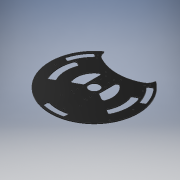
# Autodesk Inventor part: 2nd Plate
Saved by Autodesk Inventor 2017 (Build 210142000, 142)
## iProperties
Created: 2019-02-08
Part Number: 2nd Plate
Material: Generic
Document SubType Name: Modeling
Designer: cresswnd
Density: 1 g/cm^3
Appearance: Smooth - Black
Author: cresswnd
Autodesk Inventor part; units mm, degrees
ref_plane "YZ Plane" through (0, 0, 0) normal (1, 0, 0) x (0, 1, 0)
ref_plane "XZ Plane" through (0, 0, 0) normal (0, 1, 0) x (-1, 0, 0)
ref_plane "XY Plane" through (0, 0, 0) normal (0, 0, 1) x (1, 0, 0)
sketch "Sketch1" plane through (0, 0, 0) normal (0, 0, 1) x (1, 0, 0)
  circle A0 centre (21.75, 0.25) radius 1.45
  circle A1 centre (2.9989, 0.2602) radius 1.45
  circle A2 centre (-63.3205, 115.128) radius 1.45
  circle A3 centre (-53.9516, 131.369) radius 1.45
  circle A4 centre (78.6938, 131.3651) radius 1.45
  circle A5 centre (88.0766, 115.131) radius 1.45
  arc A6 (-37.626, 149.9172) -> (62.3772, 149.9149) centre (12.3777, 242.2475) ccw
  arc A7 (62.3772, 149.9149) -> (73.2296, 167.818) centre (52.5063, 168.1391) ccw
  arc A8 (-48.4787, 167.8183) -> (-37.626, 149.9172) centre (-27.7565, 168.1409) ccw
  arc A9 (-48.4787, 167.8183) -> (73.2296, 167.818) centre (12.3752, 82.2503) ccw
  circle A10 centre (12.3748, 82.2511) radius 100.0002 construction
  circle A11 centre (12.375, 82.2501) radius 12.5
  circle A12 centre (12.375, 82.2501) radius 87.5 construction
  line L0 (37.3748, -14.5737) -> (37.375, -1.6024) construction
  line L1 (-12.6233, -14.5742) -> (-12.6233, -1.603) construction
  line L2 (12.375, 82.2501) -> (114, 140.9233) construction
  line L3 (12.375, 82.2501) -> (-89.25, 140.9233) construction
  line L4 (108.7278, 109.0117) -> (97.4935, 102.5256) construction
  line L5 (83.7281, 152.3135) -> (72.4935, 145.827) construction
  arc A13 (108.7278, 109.0117) -> (83.7281, 152.3135) centre (12.3747, 82.2511) ccw
  arc A14 (97.4935, 102.5256) -> (72.4935, 145.827) centre (12.375, 82.2501) ccw
  line L6 (97.4935, 102.5256) -> (108.7278, 109.0117)
  line L7 (72.4935, 145.827) -> (83.7281, 152.3135)
  line L8 (37.3748, -14.5737) -> (37.375, -1.6024)
  line L9 (-12.6233, -14.5742) -> (-12.6233, -1.603)
  arc A15 (-12.6233, -14.5742) -> (37.3748, -14.5737) centre (12.3748, 82.2511) ccw
  arc A16 (-12.6233, -1.603) -> (37.375, -1.6024) centre (12.375, 82.2501) ccw
  line L10 (-58.9785, 152.3136) -> (-47.7434, 145.827) construction
  line L11 (-83.9782, 109.012) -> (-72.7435, 102.5256) construction
  line L12 (-72.7435, 102.5256) -> (-83.9782, 109.012)
  line L13 (-47.7434, 145.827) -> (-58.9785, 152.3136)
  arc A17 (-47.7434, 145.827) -> (-72.7435, 102.5256) centre (12.375, 82.2501) ccw
  arc A18 (-58.9785, 152.3136) -> (-83.9782, 109.012) centre (12.3717, 82.2529) ccw
  arc A19 (86.7944, 117.8432) -> (89.1811, 112.3417) centre (88.0766, 115.131) ccw
  arc A20 (76.8399, 133.7237) -> (80.4092, 128.9039) centre (78.6938, 131.3651) ccw
  arc A21 (-55.6661, 128.9072) -> (-52.0944, 133.725) centre (-53.9516, 131.369) ccw
  arc A22 (-64.4413, 112.3452) -> (-62.0519, 117.8466) centre (-63.3205, 115.128) ccw
  arc A23 (24.7176, 0.6894) -> (18.7605, -0.0012) centre (21.75, 0.25) ccw
  arc A24 (5.9875, -0.0016) -> (0.0284, 0.6799) centre (2.9989, 0.2602) ccw
  arc A25 (5.9875, -0.0016) -> (18.7605, -0.0012) centre (12.3717, 82.2529) ccw
  arc A26 (5.9875, -0.0016) -> (18.7605, -0.0012) centre (12.3717, 82.2529) ccw construction
  arc A27 (-42.373, 143.9641) -> (-52.0944, 133.725) centre (12.3717, 82.2529) ccw
  arc A28 (-36.0176, 149.0641) -> (-52.0944, 133.725) centre (12.3717, 82.2529) ccw construction
  arc A29 (-55.6661, 128.9072) -> (-62.0519, 117.8466) centre (12.3717, 82.2529) ccw
  arc A30 (-55.6661, 128.9072) -> (-62.0519, 117.8466) centre (12.3717, 82.2529) ccw construction
  arc A31 (76.8399, 133.7237) -> (67.1202, 143.9618) centre (12.3717, 82.2529) ccw
  arc A32 (76.8399, 133.7237) -> (60.7668, 149.0608) centre (12.3717, 82.2529) ccw construction
  arc A33 (86.7944, 117.8432) -> (80.4092, 128.9039) centre (12.3717, 82.2529) ccw
  arc A34 (24.7176, 0.6894) -> (89.1811, 112.3417) centre (12.3717, 82.2529) ccw construction
  arc A35 (86.7944, 117.8432) -> (80.4092, 128.9039) centre (12.3717, 82.2529) ccw construction
  line L14 (12.3717, 82.2529) -> (-95.0009, 20.2559) construction
  line L15 (12.3717, 82.2529) -> (12.3717, -55.9971) construction
  line L16 (12.3717, 82.2529) -> (116.9996, 21.845) construction
  arc A36 (-5.1266, 121.5334) -> (29.8753, 121.5311) centre (12.3717, 82.2529) ccw
  arc A37 (51.9253, 136.9246) -> (67.1202, 143.9618) centre (12.3752, 242.2457) ccw
  arc A38 (-42.373, 143.9641) -> (-27.1754, 136.9252) centre (12.3752, 242.2457) ccw
  line L17 (-23.6173, 58.5837) -> (-26.1173, 62.9138) construction
  line L18 (-26.1173, 62.9138) -> (-23.3483, 64.5125) construction
  line L19 (-23.6173, 58.5837) -> (-19.3458, 61.3318) construction
  line L20 (-23.5558, 58.6232) -> (2.0509, 58.6232) construction
  line L21 (-26.0543, 62.9502) -> (-3.8755, 75.7551)
  line L22 (-26.0543, 62.9502) -> (-0.4444, 62.9502) construction
  line L23 (12.3717, 82.2529) -> (-5.1266, 82.2529) construction
  line L24 (-5.1266, 82.2529) -> (-5.1266, 121.5334) construction
  line L25 (12.3717, 82.2529) -> (29.8753, 82.2529) construction
  line L26 (29.8753, 82.2529) -> (29.8753, 121.5311) construction
  line L27 (-5.1266, 82.2529) -> (-5.1266, 121.5334)
  line L28 (29.8753, 82.2529) -> (29.8753, 121.5311)
  line L29 (12.3717, 82.2529) -> (12.3717, 39.2511) construction
  line L30 (12.3717, 39.2511) -> (9.8717, 39.2511) construction
  line L31 (9.8717, 39.2511) -> (14.8717, 39.2511) construction
  line L32 (14.8717, 39.2511) -> (14.8717, 73.0001) construction
  line L33 (9.8717, 39.2511) -> (9.8717, 67.5643) construction
  line L34 (49.6122, 60.7517) -> (48.3622, 58.5867) construction
  line L35 (48.3622, 58.5867) -> (50.8622, 62.9168) construction
  line L36 (48.3622, 58.5867) -> (35.5366, 66.0323) construction
  line L37 (50.8622, 62.9168) -> (37.9999, 70.343) construction
  line L38 (50.7993, 62.9532) -> (28.6248, 75.7558)
  line L39 (3.3397, 3.2408) -> (3.3397, 15.3889)
  line L40 (3.3397, 3.2408) -> (15.4879, 3.2408) construction
  line L41 (21.4045, 3.23) -> (21.4045, 15.389)
  line L42 (21.4045, 3.23) -> (33.5635, 3.23) construction
  line L43 (-60.5689, 113.9329) -> (-50.0555, 107.863)
  line L44 (-60.5689, 113.9329) -> (-48.4291, 113.9329) construction
  line L45 (-51.5416, 129.5823) -> (-41.0226, 123.5092)
  line L46 (-51.5416, 129.5823) -> (-39.3953, 129.5823) construction
  line L47 (85.3244, 113.937) -> (74.8028, 107.8624)
  line L48 (85.3244, 113.937) -> (97.4738, 113.937) construction
  line L49 (76.2829, 129.5797) -> (65.7697, 123.5099)
  line L50 (76.2829, 129.5797) -> (88.4226, 129.5797) construction
  line L51 (-59.0714, 41.0016) -> (-57.8213, 38.8366) construction
  line L52 (-57.8213, 38.8366) -> (-60.3215, 43.1666) construction
  line L53 (-60.3215, 43.1666) -> (-52.3765, 47.7536) construction
  line L54 (-60.3215, 43.1666) -> (-51.1474, 43.1666) construction
  line L55 (-57.8213, 38.8366) -> (-51.421, 42.5318) construction
  line L56 (-57.8213, 38.8366) -> (-50.4308, 38.8366) construction
  line L57 (-57.7923, 38.8533) -> (-44.7683, 46.3728)
  line L58 (-57.7923, 38.8533) -> (-42.7534, 38.8533) construction
  line L59 (-60.2887, 43.1855) -> (-47.2728, 50.7003)
  line L60 (-60.2887, 43.1855) -> (-45.2593, 43.1855) construction
  line L61 (83.8121, 41.0061) -> (85.0621, 43.1712) construction
  line L62 (85.0621, 43.1712) -> (82.5621, 38.8411) construction
  line L63 (82.5621, 38.8411) -> (77.0249, 41.5028) construction
  line L64 (85.0621, 43.1712) -> (78.2875, 46.486) construction
  line L65 (82.5278, 38.8576) -> (69.5116, 46.3725)
  line L66 (82.5278, 38.8576) -> (97.5576, 38.8576) construction
  line L67 (85.0281, 43.1878) -> (72.0191, 50.6986)
  line L68 (85.0281, 43.1878) -> (100.0495, 43.1878) construction
  arc A39 (72.0191, 50.6986) -> (51.9253, 136.9246) centre (12.3717, 82.2529) ccw
  arc A40 (72.0191, 50.6986) -> (43.6909, 142.024) centre (12.3717, 82.2529) ccw construction
  arc A41 (24.7176, 0.6894) -> (82.5278, 38.8576) centre (12.3717, 82.2529) ccw
  arc A42 (85.0281, 43.1878) -> (89.1811, 112.3417) centre (12.3717, 82.2529) ccw
  arc A43 (-64.4413, 112.3452) -> (-60.2887, 43.1855) centre (12.3717, 82.2529) ccw construction
  arc A44 (-57.7923, 38.8533) -> (0.0284, 0.6799) centre (12.3717, 82.2529) ccw construction
  arc A45 (-64.4413, 112.3452) -> (-60.2887, 43.1855) centre (12.3717, 82.2529) ccw
  arc A46 (-57.7923, 38.8533) -> (0.0284, 0.6799) centre (12.3717, 82.2529) ccw
  arc A47 (-27.1754, 136.9252) -> (-47.2728, 50.7003) centre (12.3717, 82.2529) ccw
  arc A48 (-44.7683, 46.3728) -> (69.5116, 46.3725) centre (12.3717, 82.2529) ccw
  arc A49 (-5.1266, 82.2529) -> (-3.8755, 75.7551) centre (12.3717, 82.2529) ccw
  arc A50 (28.6248, 75.7558) -> (29.8753, 82.2529) centre (12.3717, 82.2529) ccw
  point P0 (-1.375, 71.4247)
  point P1 (9.8717, 39.3238)
  point P2 (9.8717, 64.9294)
  point P3 (14.8717, 39.3238)
  point P4 (14.8717, 64.9296)
  point P5 (48.2993, 58.6232)
  point P6 (26.1537, 71.4793)
  dimension "d0" = 25
  dimension "d1" = 175
  dimension "d15" = 6
  dimension "d16" = 6
  dimension "d17" = 6
  dimension "d18" = 6
  dimension "d19" = 6
  dimension "d20" = 6
  dimension "d31" = 5
  dimension "d33" = 30
  dimension "d34" = 2.5
  dimension "d35" = 5
  dimension "d36" = 2.5
  dimension "d37" = 5
  dimension "d38" = 90
  dimension "d39" = 90
  dimension "d40" = 30
  dimension "d41" = 30
  dimension "d42" = 150
  dimension "d43" = 150
  dimension "d44" = 2.5
  dimension "d45" = 5
  dimension "d46" = 30
  dimension "d47" = 30
  dimension "d48" = 30
  dimension "d49" = 30
  dimension "d50" = 2.5
  dimension "d51" = 5
  dimension "d52" = 150
  dimension "d53" = 150
  constraints: 138 end point, 115 point on circle, 50 centre point, 22 point on line, 18 horizontal, 13 coincident, 13 equal length, 7 perpendicular, 6 collinear, 5 tangent, 3 vertical, 2 concentric, 1 parallel, 13 other
  measures "d0" diameter of A11
  measures "d1" diameter of A12
  measures "d15" diameter of A19
  measures "d16" diameter of A20
  measures "d17" diameter of A21
  measures "d18" diameter of A22
  measures "d19" diameter of A23
  measures "d20" diameter of A24
  measures "d31" distance of L17.start L17.end
  measures "d33" angle of L22 L21
  measures "d34" distance of L29.end L30.end
  measures "d35" distance of L30.end L31.end
  measures "d36" distance of L34.start L34.end
  measures "d37" distance of L34.end L35.end
  measures "d38" angle of L40 L39
  measures "d39" angle of L42 L41
  measures "d40" angle of L43 L44
  measures "d41" angle of L45 L46
  measures "d42" angle of L47 L48
  measures "d43" angle of L49 L50
  measures "d44" distance of L51.start L51.end
  measures "d45" distance of L51.end L52.end
  measures "d46" angle of L54 L53
  measures "d47" angle of L56 L55
  measures "d48" angle of L58 L57
  measures "d49" angle of L60 L59
  measures "d50" distance of L61.start L61.end
  measures "d51" distance of L61.end L62.end
  measures "d52" angle of L66 L65
  measures "d53" angle of L68 L67
extrude "Extrusion4" add sketch "Sketch1" along normal blind 2 contours A6 A7 A9 A8 | A19 L47 A39 L49 A20 A33 | A21 L45 A47 L43 A22 A29 | A23 A25 A24 L39 A48 L41
fillet "Fillet1" radius 5 6 edges at (28.6248, 75.7558, 1) (50.7993, 62.9532, 1) (29.8753, 121.5311, 1) (-5.1266, 121.5334, 1) (-3.8755, 75.7551, 1) (-26.0543, 62.9502, 1)
fillet "Fillet2" radius 2 30 edges at (-51.5416, 129.5823, 1) (-52.0944, 133.725, 1) (-42.373, 143.9641, 1) (-27.1754, 136.9252, 1) (-41.0226, 123.5092, 1) (51.9253, 136.9246, 1) (67.1202, 143.9618, 1) (76.8399, 133.7237, 1) (76.2829, 129.5797, 1) (65.7697, 123.5099, 1) (89.1811, 112.3417, 1) (85.3244, 113.937, 1) (85.0281, 43.1878, 1) (72.0191, 50.6986, 1) (74.8028, 107.8624, 1) (21.4045, 15.389, 1) (21.4045, 3.23, 1) (24.7176, 0.6894, 1) (82.5278, 38.8576, 1) (69.5116, 46.3725, 1) (-60.5689, 113.9329, 1) (-64.4413, 112.3452, 1) (-50.0555, 107.863, 1) (-47.2728, 50.7003, 1) (-60.2887, 43.1855, 1) (-57.7923, 38.8533, 1) (-44.7683, 46.3728, 1) (3.3397, 3.2408, 1) (0.0284, 0.6799, 1) (3.3397, 15.3889, 1)
fillet "Fillet3" radius 3 12 edges at (37.3748, -14.5737, 1) (-12.6233, -14.5742, 1) (-12.6233, -1.603, 1) (37.375, -1.6024, 1) (-58.9785, 152.3136, 1) (-72.7435, 102.5256, 1) (-47.7434, 145.827, 1) (-83.9782, 109.012, 1) (72.4935, 145.827, 1) (83.7281, 152.3135, 1) (108.7278, 109.0117, 1) (97.4935, 102.5256, 1)
sketch "Sketch3" plane through (0, 0, 2) normal (0, 0, 1) x (1, 0, 0)
  circle A0 centre (12.375, 82.2501) radius 12.5 projected
  line L0 (12.375, 82.2501) -> (-0.7065, 69.1686) construction
  line L1 (12.375, 82.2501) -> (30.875, 82.2501) construction
  circle A1 centre (-0.7065, 69.1686) radius 1.5
  line L2 (12.375, 82.2501) -> (25.4565, 69.1686) construction
  line L3 (12.375, 82.2501) -> (30.875, 82.2501) construction
  line L4 (12.375, 82.2501) -> (25.4565, 95.3316) construction
  line L5 (12.375, 82.2501) -> (30.875, 82.2501) construction
  line L6 (12.375, 82.2501) -> (-0.7065, 95.3316) construction
  line L7 (12.375, 82.2501) -> (30.875, 82.2501) construction
  circle A2 centre (25.4565, 69.1686) radius 1.5
  circle A3 centre (25.4565, 95.3316) radius 1.5
  circle A4 centre (-0.7065, 95.3316) radius 1.5
  point P0 (0, 0)
  dimension "d66" = 18.5
  dimension "d67" = 135
  dimension "d68" = 3
  dimension "d69" = 18.5
  dimension "d70" = 45
  dimension "d71" = 18.5
  dimension "d72" = 45
  dimension "d73" = 18.5
  dimension "d74" = 135
  dimension "d75" = 3
  dimension "d76" = 3
  dimension "d77" = 3
  constraints: 16 end point, 4 centre point, 4 coincident, 4 equal length, 4 horizontal
  measures "d66" distance of L0.start L0.end
  measures "d67" angle of L0 L1
  measures "d68" diameter of A1
  measures "d69" distance of L0.start L2.end
  measures "d70" angle of L2 L3
  measures "d71" distance of L0.start L4.end
  measures "d72" angle of L5 L4
  measures "d73" distance of L0.start L6.end
  measures "d74" angle of L7 L6
  measures "d75" diameter of A2
  measures "d76" diameter of A3
  measures "d77" diameter of A4
extrude "Extrusion5" cut sketch "Sketch3" against normal up to next contours A1 | A2 | A3 | A4
sketch "Sketch4" plane through (0, 0, 2) normal (0, 0, 1) x (1, 0, 0)
  line L0 (29.8718, 12.8175) -> (-5.1282, 12.8175)
  line L1 (29.8718, 12.8175) -> (29.8718, 41.3175)
  line L2 (29.8718, 41.3175) -> (-5.1282, 41.3175)
  line L3 (-5.1282, 41.3175) -> (-5.1282, 12.8175)
  line L4 (29.8718, 27.0675) -> (34.8718, 27.0675) construction
  circle A0 centre (34.8718, 27.0675) radius 1.5 construction
  circle A1 centre (34.8718, 27.0675) radius 1.5
  line L5 (-5.1282, 27.0675) -> (-10.1282, 27.0675) construction
  circle A2 centre (-10.1282, 27.0675) radius 1.5
  line L6 (-5.1282, 41.3175) -> (-0.1282, 41.3175)
  line L7 (-0.1282, 41.3175) -> (-0.1282, 46.3175) construction
  circle A3 centre (-0.1282, 46.3175) radius 1.5
  line L8 (29.8718, 41.3175) -> (24.8718, 41.3175)
  circle A4 centre (24.8718, 46.3175) radius 1.5
  line L9 (24.8718, 46.3175) -> (24.8718, 41.3175) construction
  line L10 (-0.1282, 46.3175) -> (-0.1282, 41.3175) construction
  point P0 (0, 0)
  dimension "d88" = 35
  dimension "d89" = 28.5
  dimension "d93" = 5
  dimension "d94" = 3
  dimension "d95" = 5
  dimension "d96" = 3
  dimension "d101" = 5
  dimension "d102" = 5
  dimension "d103" = 3
  dimension "d104" = 5
  dimension "d106" = 3
  constraints: 22 end point, 5 centre point, 4 coincident, 3 perpendicular, 2 horizontal, 2 midpoint, 2 point on line, 2 vertical, 1 collinear, 1 concentric
  measures "d88" distance of L0.start L0.end
  measures "d89" distance of L0.start L1.end
  measures "d93" distance of L4.start L4.end
  measures "d94" diameter of A0
  measures "d95" distance of L5.start L5.end
  measures "d96" diameter of A2
  measures "d101" distance of L2.end L6.end
  measures "d102" distance of L6.end L7.end
  measures "d103" diameter of A3
  measures "d104" distance of L1.end L8.end
  measures "d106" diameter of A4
fillet "Fillet4" radius 1 2 edges at (-48.4787, 167.8183, 1) (73.2296, 167.818, 1)
extrude "Extrusion7" cut sketch "Sketch4" against normal up to next contours A1 | A2 | A3 | A4
sketch "Sketch5" plane through (0, 0, 2) normal (0, 0, 1) x (1, 0, 0)
  circle A0 centre (12.375, 82.2501) radius 12.5 construction
  line L0 (12.375, 82.2501) -> (142.3592, 82.2501) construction
  line L1 (12.375, 82.2501) -> (-110.5194, 82.2501) construction
  arc A1 (86.0051, 45.0622) -> (89.7572, 110.8276) centre (12.3717, 82.2529) ccw construction
  line L2 (94.8643, 82.2501) -> (104.8643, 82.2501) construction
  arc A2 (-65.0201, 110.8238) -> (-61.2657, 45.0599) centre (12.3717, 82.2529) ccw construction
  line L3 (-70.1255, 82.2501) -> (-80.1255, 82.2501) construction
  circle A3 centre (104.8643, 82.2501) radius 1.5
  circle A4 centre (-80.1255, 82.2501) radius 1.5
  point P0 (0, 0)
  dimension "d109" = 10
  dimension "d110" = 10
  dimension "d111" = 3
  dimension "d112" = 3
  constraints: 8 end point, 4 point on line, 2 centre point, 2 coincident, 2 horizontal, 2 point on circle
  measures "d109" distance of L2.start L2.end
  measures "d110" distance of L3.start L3.end
  measures "d111" diameter of A3
  measures "d112" diameter of A4
extrude "Extrusion8" cut sketch "Sketch5" against normal up to next
sketch "Sketch8" plane through (0, 0, 2) normal (0, 0, 1) x (1, 0, 0)
  circle A0 centre (29.8754, 127.8011) radius 1.5 projected
  circle A1 centre (-5.1266, 127.8012) radius 1.5 projected
  point P0 (0, 0)
extrude "Extrusion11" cut sketch "Sketch8" against normal up to next
sketch "Sketch9" plane through (0, 0, 0) normal (0, 0, -1) x (-1, 0, 0)
  circle A0 centre (-12.375, 82.2501) radius 12.5 projected
  line L0 (-12.375, 82.2501) -> (5.1266, 82.2529) construction
  line L1 (5.1266, 82.2529) -> (0.125, 82.2521) construction
  circle A1 centre (-12.375, 82.2501) radius 12.5 construction
  circle A2 centre (2.6258, 82.2525) radius 1.5
  line L2 (-12.375, 82.2501) -> (-12.375, 78) construction
  circle A3 centre (-27.3758, 82.2525) radius 1.5
  line L3 (-12.375, 82.2501) -> (-12.375, 159) construction
  arc A4 (-62.3772, 149.9149) -> (37.626, 149.9172) centre (-12.3777, 242.2475) ccw construction
  line L4 (-12.3753, 137.2463) -> (-12.375, 119.7463) construction
  line L5 (-12.375, 119.7463) -> (-2.875, 119.7463) construction
  circle A5 centre (-2.875, 119.7463) radius 1.5
  circle A6 centre (-21.875, 119.7463) radius 1.5
  circle A7 centre (0.1282, 46.3175) radius 1.5 construction
  line L6 (0.1282, 46.3175) -> (0.1282, 69.1686) construction
  circle A8 centre (-24.8718, 46.3175) radius 1.5 construction
  line L7 (-24.8718, 46.3175) -> (-24.8718, 69.1686) construction
  line L8 (0.1282, 57.7431) -> (8, 57.7431) construction
  line L9 (2.6258, 82.2525) -> (2.6258, 57.7431) construction
  circle A9 centre (2.6258, 57.7431) radius 1.5
  circle A10 centre (-27.3758, 57.7431) radius 1.5
  circle A11 centre (-2.875, 107.2463) radius 1.5
  line L10 (-2.875, 107.2463) -> (-2.875, 119.7463) construction
  circle A12 centre (-21.875, 107.2463) radius 1.5
  point P0 (0, 0)
  dimension "d121" = 3
  dimension "d122" = 17.5
  dimension "d123" = 9.5
  dimension "d124" = 3
  dimension "d125" = 3
  dimension "d127" = 3
  dimension "d130" = 12.5
  constraints: 22 end point, 8 centre point, 4 symmetric about line, 4 vertical, 3 point on line, 2 coincident, 2 horizontal, 2 midpoint, 2 perpendicular, 1 point on circle, 6 other
  measures "d121" diameter of A2
  measures "d122" distance of L4.start L4.end
  measures "d123" distance of L4.end L5.end
  measures "d124" diameter of A5
  measures "d125" diameter of A9
  measures "d127" diameter of A11
  measures "d130" distance of L10.start L10.end
extrude "Extrusion12" cut sketch "Sketch9" against normal up to next contours A2 | A3 | A5 | A6 | A9 | A10 | A11 | A12
sketch "Sketch12" plane through (0, 0, 0) normal (0, 0, -1) x (-1, 0, 0)
  circle A0 centre (-2.875, 107.2463) radius 1.5 projected
  circle A1 centre (2.6258, 57.7431) radius 1.5 projected
  circle A2 centre (-2.875, 119.7463) radius 1.5 projected
  circle A3 centre (2.6258, 82.2525) radius 1.5 projected
  circle A4 centre (-27.3758, 82.2525) radius 1.5 projected
  circle A5 centre (-21.875, 119.7463) radius 1.5 projected
  circle A6 centre (-27.3758, 57.7431) radius 1.5 projected
  circle A7 centre (-21.875, 107.2463) radius 1.5 projected
  circle A8 centre (-29.8754, 127.8011) radius 1.5 projected
  circle A9 centre (5.1266, 127.8012) radius 1.5 projected
  circle A10 centre (-104.8643, 82.2501) radius 1.5 projected
  circle A11 centre (80.1255, 82.2501) radius 1.5 projected
  circle A12 centre (0.1282, 46.3175) radius 1.5 projected
  circle A13 centre (-34.8718, 27.0675) radius 1.5 projected
  circle A14 centre (10.1282, 27.0675) radius 1.5 projected
  circle A15 centre (-24.8718, 46.3175) radius 1.5 projected
  circle A16 centre (-25.4565, 95.3316) radius 1.5 projected
  circle A17 centre (0.7065, 69.1686) radius 1.5 projected
  circle A18 centre (-25.4565, 69.1686) radius 1.5 projected
  circle A19 centre (0.7065, 95.3316) radius 1.5 projected
  arc A20 (28.3785, 68.5207) -> (13.0868, 116.9085) centre (-12.3717, 82.2529) ccw projected
  arc A21 (21.1403, 65.7873) -> (28.3785, 68.5207) centre (23.6403, 70.1174) ccw projected
  line L0 (21.1403, 65.7873) -> (7.2472, 73.8084) projected
  arc A22 (4.8316, 79.0529) -> (7.2472, 73.8084) centre (9.7472, 78.1385) ccw projected
  arc A23 (4.8316, 79.0529) -> (5.1266, 82.2529) centre (-12.3717, 82.2529) ccw projected
  line L1 (5.1266, 82.2529) -> (5.1266, 112.879) projected
  arc A24 (13.0868, 116.9085) -> (5.1266, 112.879) centre (10.1266, 112.879) ccw projected
  line L2 (-31.9961, 73.8093) -> (-45.8848, 65.7905) projected
  arc A25 (-53.1232, 68.5244) -> (-45.8848, 65.7905) centre (-48.3849, 70.1207) ccw projected
  arc A26 (-37.8361, 116.9042) -> (-53.1232, 68.5244) centre (-12.3717, 82.2529) ccw projected
  arc A27 (-29.8753, 112.8752) -> (-37.8361, 116.9042) centre (-34.8753, 112.8752) ccw projected
  line L3 (-29.8753, 112.8752) -> (-29.8753, 82.2529) projected
  arc A28 (-29.8753, 82.2529) -> (-29.5804, 79.0534) centre (-12.3717, 82.2529) ccw projected
  arc A29 (-31.9961, 73.8093) -> (-29.5804, 79.0534) centre (-34.4961, 78.1394) ccw projected
  arc A30 (1.5791, 0.9393) -> (56.6574, 37.07) centre (-12.3717, 82.2529) ccw projected
  arc A31 (-0.455, 1.8504) -> (1.5791, 0.9393) centre (1.2409, 2.9105) ccw projected
  arc A32 (-0.455, 1.8504) -> (-2.0034, 3.0903) centre (-2.9989, 0.2602) ccw projected
  arc A33 (-3.3397, 4.9769) -> (-2.0034, 3.0903) centre (-1.3397, 4.9769) ccw projected
  line L4 (-3.3397, 4.9769) -> (-3.3397, 13.6632) projected
  arc A34 (-1.6573, 15.6378) -> (-3.3397, 13.6632) centre (-1.3397, 13.6632) ccw projected
  arc A35 (-1.6573, 15.6378) -> (43.7504, 44.8007) centre (-12.3717, 82.2529) ccw projected
  arc A36 (46.414, 45.4226) -> (43.7504, 44.8007) centre (45.414, 43.6905) ccw projected
  line L5 (46.414, 45.4226) -> (55.984, 39.8974) projected
  arc A37 (56.6574, 37.07) -> (55.984, 39.8974) centre (54.984, 38.1653) ccw projected
  arc A38 (61.3674, 112.8509) -> (63.2145, 112.1299) centre (63.3205, 115.128) ccw projected
  arc A39 (65.0201, 110.8238) -> (63.2145, 112.1299) centre (63.1439, 110.1311) ccw projected
  arc A40 (61.2657, 45.0599) -> (65.0201, 110.8238) centre (-12.3717, 82.2529) ccw projected
  arc A41 (58.4805, 44.2295) -> (61.2657, 45.0599) centre (59.4805, 45.9616) ccw projected
  line L6 (58.4805, 44.2295) -> (48.9187, 49.75) projected
  arc A42 (48.1256, 52.3678) -> (48.9187, 49.75) centre (49.9187, 51.482) ccw projected
  arc A43 (48.1256, 52.3678) -> (50.6811, 106.2816) centre (-12.3717, 82.2529) ccw projected
  arc A44 (51.55, 108.7258) -> (50.6811, 106.2816) centre (52.55, 106.9938) ccw projected
  line L7 (51.55, 108.7258) -> (59.0653, 113.0648) projected
  arc A45 (61.3674, 112.8509) -> (59.0653, 113.0648) centre (60.0653, 111.3328) ccw projected
  arc A46 (-22.7427, 3.081) -> (-24.287, 1.8512) centre (-21.75, 0.25) ccw projected
  arc A47 (-26.3163, 0.9475) -> (-24.287, 1.8512) centre (-25.9783, 2.9187) ccw projected
  arc A48 (-81.3928, 37.0742) -> (-26.3163, 0.9475) centre (-12.3717, 82.2529) ccw projected
  arc A49 (-80.7194, 39.9016) -> (-81.3928, 37.0742) centre (-79.7194, 38.1696) ccw projected
  line L8 (-80.7194, 39.9016) -> (-71.1573, 45.4223) projected
  arc A50 (-68.4937, 44.8004) -> (-71.1573, 45.4223) centre (-70.1573, 43.6903) ccw projected
  arc A51 (-68.4937, 44.8004) -> (-23.0869, 15.638) centre (-12.3717, 82.2529) ccw projected
  arc A52 (-21.4045, 13.6633) -> (-23.0869, 15.638) centre (-23.4045, 13.6633) ccw projected
  line L9 (-21.4045, 13.6633) -> (-21.4045, 4.9683) projected
  arc A53 (-22.7427, 3.081) -> (-21.4045, 4.9683) centre (-23.4045, 4.9683) ccw projected
  arc A54 (-89.7572, 110.8276) -> (-86.0051, 45.0622) centre (-12.3717, 82.2529) ccw projected
  arc A55 (-87.9592, 112.1333) -> (-89.7572, 110.8276) centre (-87.881, 110.1348) ccw projected
  arc A56 (-87.9592, 112.1333) -> (-86.1229, 112.8544) centre (-88.0766, 115.131) ccw projected
  arc A57 (-83.8204, 113.0687) -> (-86.1229, 112.8544) centre (-84.8204, 111.3366) ccw projected
  line L10 (-83.8204, 113.0687) -> (-76.2972, 108.7252) projected
  arc A58 (-75.4283, 106.281) -> (-76.2972, 108.7252) centre (-77.2972, 106.9931) ccw projected
  arc A59 (-75.4283, 106.281) -> (-72.8719, 52.3662) centre (-12.3717, 82.2529) ccw projected
  arc A60 (-73.665, 49.7483) -> (-72.8719, 52.3662) centre (-74.665, 51.4804) ccw projected
  line L11 (-73.665, 49.7483) -> (-83.2199, 44.2318) projected
  arc A61 (-86.0051, 45.0622) -> (-83.2199, 44.2318) centre (-84.2199, 45.9639) ccw projected
  arc A62 (71.7645, 106.2666) -> (50.4937, 143.1087) centre (-12.375, 82.2501) ccw projected
  arc A63 (51.1492, 147.7934) -> (50.4937, 143.1087) centre (52.6492, 145.1953) ccw projected
  line L12 (51.1492, 147.7934) -> (56.9413, 151.1374) projected
  arc A64 (60.6314, 150.5895) -> (56.9413, 151.1374) centre (58.4413, 148.5393) ccw projected
  arc A65 (83.3116, 111.3055) -> (60.6314, 150.5895) centre (-12.3717, 82.2529) ccw projected
  arc A66 (81.941, 107.8358) -> (83.3116, 111.3055) centre (80.441, 110.4339) ccw projected
  line L13 (81.941, 107.8358) -> (76.1493, 104.4919) projected
  arc A67 (71.7645, 106.2666) -> (76.1493, 104.4919) centre (74.6493, 107.09) ccw projected
  line L14 (-100.8993, 104.492) -> (-106.6906, 107.8356) projected
  arc A68 (-108.0612, 111.3053) -> (-106.6906, 107.8356) centre (-105.1906, 110.4337) ccw projected
  arc A69 (-85.3811, 150.5894) -> (-108.0612, 111.3053) centre (-12.3747, 82.2511) ccw projected
  arc A70 (-81.6909, 151.1373) -> (-85.3811, 150.5894) centre (-83.1909, 148.5392) ccw projected
  line L15 (-81.6909, 151.1373) -> (-75.8992, 147.7933) projected
  arc A71 (-75.2438, 143.1087) -> (-75.8992, 147.7933) centre (-77.3993, 145.1953) ccw projected
  arc A72 (-75.2438, 143.1087) -> (-96.5145, 106.2666) centre (-12.375, 82.2501) ccw projected
  arc A73 (-100.8993, 104.492) -> (-96.5145, 106.2666) centre (-99.3993, 107.0901) ccw projected
  arc A74 (-35.0553, -15.1431) -> (10.3036, -15.1436) centre (-12.3748, 82.2511) ccw projected
  arc A75 (-37.3749, -12.2213) -> (-35.0553, -15.1431) centre (-34.3749, -12.2213) ccw projected
  line L16 (-37.3749, -12.2213) -> (-37.375, -5.5352) projected
  arc A76 (-33.6457, -2.6251) -> (-37.375, -5.5352) centre (-34.375, -5.5352) ccw projected
  arc A77 (-33.6457, -2.6251) -> (8.894, -2.6256) centre (-12.375, 82.2501) ccw projected
  arc A78 (12.6233, -5.5356) -> (8.894, -2.6256) centre (9.6233, -5.5356) ccw projected
  line L17 (12.6233, -5.5356) -> (12.6233, -12.2218) projected
  arc A79 (10.3036, -15.1436) -> (12.6233, -12.2218) centre (9.6233, -12.2218) ccw projected
  circle A80 centre (-12.375, 82.2501) radius 12.5 projected
  arc A81 (-75.7452, 130.8123) -> (-76.0427, 132.7692) centre (-78.6938, 131.3651) ccw projected
  arc A82 (-75.8134, 134.9837) -> (-76.0427, 132.7692) centre (-74.2753, 133.7053) ccw projected
  arc A83 (-68.1888, 142.9969) -> (-75.8134, 134.9837) centre (-12.3717, 82.2529) ccw projected
  arc A84 (-65.8843, 143.2835) -> (-68.1888, 142.9969) centre (-66.8356, 141.5242) ccw projected
  arc A85 (-65.8843, 143.2835) -> (-55.1953, 138.2112) centre (-12.3752, 242.2457) ccw projected
  arc A86 (-54.7019, 134.8042) -> (-55.1953, 138.2112) centre (-55.9565, 136.3617) ccw projected
  arc A87 (-54.7019, 134.8042) -> (-64.7129, 124.8425) centre (-12.3717, 82.2529) ccw projected
  arc A88 (-67.2643, 124.3728) -> (-64.7129, 124.8425) centre (-66.2643, 126.1048) ccw projected
  line L18 (-67.2643, 124.3728) -> (-74.7795, 128.7117) projected
  arc A89 (-75.7452, 130.8123) -> (-74.7795, 128.7117) centre (-73.7795, 130.4438) ccw projected
  arc A90 (51.069, 134.9836) -> (43.4417, 142.9992) centre (-12.3717, 82.2529) ccw projected
  arc A91 (51.2992, 132.7707) -> (51.069, 134.9836) centre (49.5309, 133.7052) ccw projected
  arc A92 (51.2992, 132.7707) -> (51.0031, 130.8152) centre (53.9516, 131.369) ccw projected
  arc A93 (50.0375, 128.7139) -> (51.0031, 130.8152) centre (49.0375, 130.446) ccw projected
  line L19 (50.0375, 128.7139) -> (42.5172, 124.3721) projected
  arc A94 (39.9659, 124.8418) -> (42.5172, 124.3721) centre (41.5172, 126.1041) ccw projected
  arc A95 (39.9659, 124.8418) -> (29.9524, 134.8048) centre (-12.3717, 82.2529) ccw projected
  arc A96 (30.4457, 138.2119) -> (29.9524, 134.8048) centre (31.2069, 136.3625) ccw projected
  arc A97 (30.4457, 138.2119) -> (41.1372, 143.2858) centre (-12.3752, 242.2457) ccw projected
  arc A98 (43.4417, 142.9992) -> (41.1372, 143.2858) centre (42.0885, 141.5265) ccw projected
  circle A99 centre (-88.0766, 115.131) radius 1.45 projected
  circle A100 centre (-78.6938, 131.3651) radius 1.45 projected
  circle A101 centre (53.9516, 131.369) radius 1.45 projected
  circle A102 centre (63.3205, 115.128) radius 1.45 projected
  circle A103 centre (-2.9989, 0.2602) radius 1.45 projected
  circle A104 centre (-21.75, 0.25) radius 1.45 projected
  arc A105 (-73.1254, 166.0393) -> (-74.714, 166.7427) centre (-74.1203, 165.938) ccw projected
  arc A106 (-74.714, 166.7427) -> (49.9629, 166.7431) centre (-12.3752, 82.2503) ccw projected
  arc A107 (49.9629, 166.7431) -> (48.3744, 166.0398) centre (49.3692, 165.9384) ccw projected
  arc A108 (37.626, 149.9172) -> (48.3744, 166.0398) centre (27.7565, 168.1409) ccw projected
  arc A109 (-62.3772, 149.9149) -> (37.626, 149.9172) centre (-12.3777, 242.2475) ccw projected
  arc A110 (-73.1254, 166.0393) -> (-62.3772, 149.9149) centre (-52.5063, 168.1391) ccw projected
  point P0 (0, 0)
extrude "Extrusion14" add sketch "Sketch12" against normal blind 2 contours A31 A32 A33 L4 A34 A35 A36 L5 A37 A30 | A46 A47 A48 A49 L8 A50 A51 A52 L9 A53 | A81 A82 A83 A84 A85 A86 A87 A88 L18 A89 | A91 A92 A93 L19 A94 A95 A96 A97 A98 A90
sketch "Sketch13" plane through (0, 0, 2) normal (0, 0, 1) x (1, 0, 0)
  arc A0 (-37.626, 149.9172) -> (62.3772, 149.9149) centre (12.3777, 242.2475) ccw projected
  arc A1 (-48.3744, 166.0398) -> (-37.626, 149.9172) centre (-27.7565, 168.1409) ccw projected
  arc A2 (-37.626, 149.9172) -> (62.3772, 149.9149) centre (12.3777, 242.2475) ccw construction
  line L0 (-56.9413, 151.1374) -> (-51.1492, 147.7934) construction
  line L1 (12.3753, 137.2463) -> (12.3753, 149.7463) construction
  arc A3 (62.3772, 149.9149) -> (73.1254, 166.0393) centre (52.5063, 168.1391) ccw construction
  line L2 (-37.3091, 149.7463) -> (-54.5317, 149.7463) construction
  line L3 (62.0645, 149.7463) -> (79.2817, 149.7463) construction
  line L4 (81.6909, 151.1373) -> (75.8992, 147.7933) construction
  line L5 (-45.9204, 149.7463) -> (-44.2103, 145.0478) construction
  line L6 (-45.9204, 149.7463) -> (-40.9204, 149.7463) construction
  circle A4 centre (-44.2103, 145.0478) radius 1.5 construction
  line L7 (70.6711, 149.7463) -> (68.961, 145.0478) construction
  circle A5 centre (68.961, 145.0478) radius 1.5 construction
  circle A6 centre (68.961, 145.0478) radius 1.5
  circle A7 centre (-44.2103, 145.0478) radius 1.5
  line L8 (70.6711, 149.7463) -> (74.5013, 152.9602)
  line L9 (70.6711, 149.7463) -> (75.6711, 149.7463) construction
  circle A8 centre (74.5013, 152.9602) radius 1.5
  line L10 (-45.9204, 149.7463) -> (-49.7507, 152.9602)
  circle A9 centre (-49.7507, 152.9602) radius 1.5
  point P0 (0, 0)
  dimension "d135" = 12.5
  dimension "d138" = 5
  dimension "d139" = 70
  dimension "d141" = 3
  dimension "d145" = 5
  dimension "d146" = 40
  dimension "d147" = 3
  constraints: 18 end point, 6 centre point, 6 coincident, 5 symmetric about line, 3 horizontal, 3 point on circle, 2 equal length, 2 point on line, 1 concentric, 1 midpoint, 1 vertical, 2 other
  measures "d135" distance of L1.start L1.end
  measures "d138" distance of L5.start L5.end
  measures "d139" angle of L5 L6
  measures "d141" diameter of A4
  measures "d145" distance of L7.start L8.end
  measures "d146" angle of L9 L8
  measures "d147" diameter of A8
extrude "Extrusion15" cut sketch "Sketch13" against normal blind 2
sketch "Sketch14" plane through (0, 0, 0) normal (0, 0, -1) x (-1, 0, 0)
  circle A0 centre (-98.8862, 32.3027) radius 1.5
  circle A1 centre (74.1362, 32.3027) radius 1.5
  circle A2 centre (-30.5525, 46.8657) radius 1.5
  circle A3 centre (5.8025, 46.8657) radius 1.5
  point P0 (0, 0)
  constraints: 4 centre point, 8 other
extrude "Extrusion16" cut sketch "Sketch14" against normal up to next
body "Solid4"
